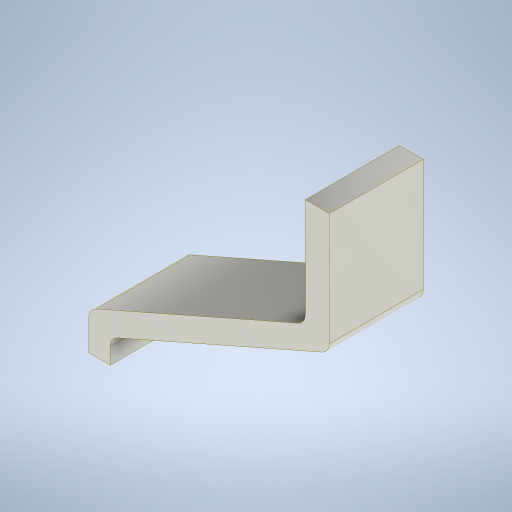
# Autodesk Inventor part: Limit switch sheet
Saved by Autodesk Inventor 2023 (Build 270158000, 158)
## iProperties
Created: 2023-12-14
Part Number: Limit switch sheet
Material: Silver
Document SubType Name: Modeling
Designer: User
Density: 10.49 g/cm^3
Appearance: Silver
Author: User
Autodesk Inventor part; units mm, degrees
ref_plane "YZ Plane" through (0, 0, 0) normal (1, 0, 0) x (0, 1, 0)
ref_plane "XZ Plane" through (0, 0, 0) normal (0, 1, 0) x (-1, 0, 0)
ref_plane "XY Plane" through (0, 0, 0) normal (0, 0, 1) x (1, 0, 0)
sketch "Sketch1" plane through (0, 0, 0) normal (0, 0, 1) x (1, 0, 0)
  line L0 (9, 0) -> (10, 0)
  line L1 (13, 0) -> (13, -10)
  line L2 (0, -13.9226) -> (0, -8.7389) construction
  line L3 (0.9, -13.9226) -> (0.9, -9.3264) construction
  line L4 (-0.7394, -10) -> (2.996, -10) construction
  line L5 (-0.7394, -9) -> (2.996, -9) construction
  line L6 (-0.7394, -5) -> (10, -5) construction
  line L7 (1.1988, -8.8687) -> (9.7012, -5.1313)
  line L8 (0.2988, -8.2812) -> (8.7012, -4.5878)
  arc A0 (0.2988, -8.2812) -> (0, -8.7389) centre (0.5, -8.7389) ccw
  arc A1 (1.1988, -8.8687) -> (0.9, -9.3264) centre (1.4, -9.3264) ccw
  line L9 (0.9, -9.3264) -> (0.9, -10)
  line L10 (0.9, -10) -> (0, -10)
  line L11 (10, 0) -> (10, -4.6736)
  line L12 (10, -13.9226) -> (10, -10) construction
  line L13 (10, -5) -> (10, 0) construction
  line L14 (9, 0) -> (9, -4.1301)
  line L15 (0, -8.7389) -> (0, -10)
  arc A2 (8.7012, -4.5878) -> (9, -4.1301) centre (8.5, -4.1301) ccw
  arc A3 (9.7012, -5.1313) -> (10, -4.6736) centre (9.5, -4.6736) ccw
  point P0 (0, 0)
  point P1 (0, -6.4341)
  point P2 (0.9, -9)
  dimension "d0" = 13
  dimension "d1" = 10
  dimension "d2" = 0.9
  dimension "d3" = 1
  dimension "d5" = 4
  dimension "d6" = 0.9
  dimension "d7" = 0.5
  dimension "d8" = 1
  dimension "d9" = 0.5
  constraints: 32 end point, 8 point on circle, 8 point on line, 8 tangent, 6 parallel, 4 centre point, 4 collinear, 2 equal radius, 1 horizontal, 1 perpendicular
  measures "d0" distance of L1.end L10.end
  measures "d1" distance of L1.start L1.end
  measures "d2" distance between parallel lines of L2 L3
  measures "d3" distance between parallel lines of L4 L5
  measures "d5" distance between parallel lines of L5 L6
  measures "d6" distance between parallel lines of L7 L8
  measures "d7" radius of A0
  measures "d8" distance between parallel lines of L11 L14
  measures "d9" radius of A2
extrude "Extrusion1" add sketch "Sketch1" along normal blind 3.9
body "Solid1"
